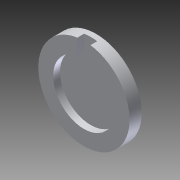
# Autodesk Inventor part: ContactPuck
Saved by Autodesk Inventor 2012 SP1 (Build 160190100, 190)
## iProperties
Created: 2010-03-11
Part Number: ContactPuck
Document SubType Name: Modeling
Designer: rconnaug
Density: 1.42 g/cm^3
Material: Acetal Resin, White
Mass: 3.30031 g
Surface Area: 18.8737 cm^2
Volume: 2.32416 cm^3
Author: rconnaug
Autodesk Inventor part; units mm, degrees
ref_plane "YZ Plane" through (0, 0, 0) normal (1, 0, 0) x (0, 1, 0)
ref_plane "XZ Plane" through (0, 0, 0) normal (0, 1, 0) x (-1, 0, 0)
ref_plane "XY Plane" through (0, 0, 0) normal (0, 0, 1) x (1, 0, 0)
sketch "Sketch1" plane through (0, 0, 0) normal (0, 0, 1) x (1, 0, 0)
  circle A0 centre (0, 0) radius 14.859
  dimension "d0" = 29.718
  constraints: 1 centre point, 1 coincident
  measures "d0" diameter of A0
extrude "Extrusion1" add sketch "Sketch1" along normal blind 3.9624
sketch "Sketch2" plane through (0, 0, 3.9624) normal (0, 0, 1) x (1, 0, 0)
  circle A0 centre (0, 0) radius 14.859 projected
  line L0 (0, -21) -> (0, 21) projected
  arc A1 (-2.125, 9.7716) -> (2.125, 9.7716) centre (0, 0) ccw
  line L1 (-2.125, 14.859) -> (2.125, 14.859)
  line L2 (2.125, 14.859) -> (2.125, 9.7716)
  line L3 (-2.125, 9.7716) -> (-2.125, 14.859)
  point P0 (0, 14.859)
  dimension "d3" = 20
  dimension "d4" = 4.25
  constraints: 6 end point, 2 point on circle, 1 centre point, 1 coincident, 1 horizontal, 1 midpoint, 1 parallel, 1 perpendicular, 1 point on line, 1 tangent
  measures "d3" diameter of A1
  measures "d4" distance of L1.start L1.end
extrude "Extrusion2" cut sketch "Sketch2" against normal blind 2.2075 contours L2 A1 L0 A0 | A0 L1 L2 | L0 A1 L3 A0 | A0 L3 L1 picked at (0.7083, 4.8769) picked at (-5.7183, -2.5578)
body "Solid1"
